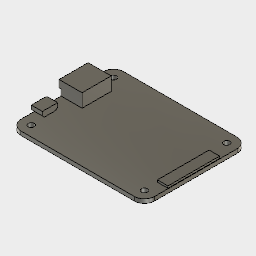
2218 HDMI TPF401 Breakout (Autodesk Fusion 360 design; units mm, degrees)
Autodesk Fusion 360 part; units mm, degrees
sketch "PCB" plane through (0, 0, 0) normal (0, 0, 1) x (1, 0, 0)
  line L0 (0, 0) -> (66.04, 0)
  line L1 (66.04, 0) -> (66.04, 50.8)
  line L2 (66.04, 50.8) -> (0, 50.8)
  line L3 (0, 50.8) -> (0, 0)
  circle A0 centre (5.08, 45.72) radius 1.5
  line L4 (33.02, 50.8) -> (33.02, 0) construction
  line L5 (0, 25.4) -> (66.04, 25.4) construction
  circle A1 centre (60.96, 45.72) radius 1.5
  circle A2 centre (5.08, 5.08) radius 1.5
  circle A3 centre (60.96, 5.08) radius 1.5
  dimension "d1" = 66.04
  dimension "d2" = 50.8
  dimension "d3" = 3
  dimension "d4" = 5.08
  dimension "d5" = 45.72
  measures "d1" distance of L1.end L2.end
  measures "d2" distance of L0.end L1.end
  measures "d3" diameter of A0
  measures "d4" distance of L3 A0.centre
  measures "d5" distance of L0 A0.centre
extrude "Extrude1" add sketch "PCB" along normal blind 2 makes body 1
fillet "Fillet1" radius 5.08 4 edges at (66.04, 0, 1) (0, 0, 1) (0, 50.8, 1) (66.04, 50.8, 1) on bodies 1
sketch "hdmi usb" plane through (0, 0, 2) normal (0, 0, 1) x (-1, 0, 0)
  arc A0 (-66.04, -45.72) -> (-60.96, -50.8) centre (-60.96, -45.72) ccw
  line L0 (-60.96, -50.8) -> (-5.08, -50.8)
  arc A1 (-5.08, -50.8) -> (0, -45.72) centre (-5.08, -45.72) ccw
  line L1 (0, -45.72) -> (0, -5.08)
  arc A2 (0, -5.08) -> (-5.08, 0) centre (-5.08, -5.08) ccw
  line L2 (-5.08, 0) -> (-60.96, 0)
  arc A3 (-60.96, 0) -> (-66.04, -5.08) centre (-60.96, -5.08) ccw
  line L3 (-66.04, -5.08) -> (-66.04, -45.72)
  circle A4 centre (-60.96, -5.08) radius 1.5
  circle A5 centre (-60.96, -45.72) radius 1.5
  circle A6 centre (-5.08, -45.72) radius 1.5
  circle A7 centre (-5.08, -5.08) radius 1.5
  line L4 (1, -39.24) -> (-10.4, -39.24)
  line L5 (-10.4, -39.24) -> (-10.4, -24.84)
  line L6 (-10.4, -24.84) -> (1, -24.84)
  line L7 (1, -24.84) -> (1, -39.24)
  line L8 (0.6, -18.34) -> (-4.9, -18.34)
  line L9 (-4.9, -18.34) -> (-4.9, -10.74)
  line L10 (-4.9, -10.74) -> (0.6, -10.74)
  line L11 (0.6, -10.74) -> (0.6, -18.34)
  dimension "d9" = 11.4
  dimension "d10" = 14.4
  dimension "d11" = 1
  dimension "d12" = 11.56
  dimension "d13" = 5.5
  dimension "d14" = 7.6
  dimension "d15" = 0.6
  dimension "d16" = 6.5
  measures "d9" distance of L4.start L4.end
  measures "d10" distance of L4.start L6.end
  measures "d11" distance of L1 L7
  measures "d12" distance of L0 L4
  measures "d13" distance of L8.start L8.end
  measures "d14" distance of L8.start L10.end
  measures "d15" distance of L1 L11
  measures "d16" distance of L6 L8
extrude "Extrude2" add sketch "hdmi usb" along normal blind 5.6 from surface at 1 separate body contours L1 L4 L5 L6 | L1 L4 L6 L7 makes body 2
chamfer "Chamfer1" distance 2 angle 45 2 edges at (4.7, 24.84, 3) (4.7, 39.24, 3) on bodies 2
extrude "Extrude3" add sketch "hdmi usb" along normal blind 2.9 separate body contours L1 L8 L10 L11 | L1 L8 L9 L10 makes body 3
chamfer "Chamfer2" distance 1 angle 45 2 edges at (2.15, 18.34, 2) (2.15, 10.74, 2) on bodies 3
sketch "hdmi 2" plane through (0, 0, 3) normal (0, 0, -1) x (1, 0, 0)
  line L0 (-1, -37.24) -> (10.4, -37.24)
  line L1 (10.4, -37.24) -> (10.4, -26.84)
  line L2 (10.4, -26.84) -> (-1, -26.84)
  line L3 (-1, -26.84) -> (-1, -37.24)
  line L4 (0, -45.72) -> (0, -5.08)
  line L5 (-1, -24.84) -> (10.4, -24.84)
  line L6 (10.4, -24.84) -> (10.4, -39.24)
  line L7 (10.4, -39.24) -> (-1, -39.24)
  line L8 (-1, -39.24) -> (-1, -24.84)
extrude "Extrude4" add sketch "hdmi 2" along normal blind 1 contours L0 L1 L2 L4 L6 bodies 2
extrude "Extrude5" add sketch "hdmi 2" along normal blind -2.5 and the other way blind -1 contours L0 L4 L6 L7 | L2 L4 L5 L6 bodies 2
sketch "Sketch4" plane through (0, 0, 2) normal (0, 0, 1) x (-1, 0, 0)
  arc A0 (-66.04, -45.72) -> (-60.96, -50.8) centre (-60.96, -45.72) ccw
  line L0 (-60.96, -50.8) -> (-5.08, -50.8)
  arc A1 (-5.08, -50.8) -> (0, -45.72) centre (-5.08, -45.72) ccw
  line L1 (0, -45.72) -> (0, -5.08)
  arc A2 (0, -5.08) -> (-5.08, 0) centre (-5.08, -5.08) ccw
  line L2 (-5.08, 0) -> (-60.96, 0)
  arc A3 (-60.96, 0) -> (-66.04, -5.08) centre (-60.96, -5.08) ccw
  line L3 (-66.04, -5.08) -> (-66.04, -45.72)
  circle A4 centre (-60.96, -5.08) radius 1.5
  circle A5 centre (-60.96, -45.72) radius 1.5
  circle A6 centre (-5.08, -45.72) radius 1.5
  circle A7 centre (-5.08, -5.08) radius 1.5
  line L4 (-60.64, -37.3) -> (-65.84, -37.3)
  line L5 (-65.84, -37.3) -> (-65.84, -11.8)
  line L6 (-65.84, -11.8) -> (-60.64, -11.8)
  line L7 (-60.64, -11.8) -> (-60.64, -37.3)
  line L8 (-60.64, -24.55) -> (-65.84, -24.55) construction
  dimension "d30" = 25.5
  dimension "d31" = 24.55
  dimension "d32" = 0.2
  dimension "d33" = 5.2
  measures "d30" distance of L4.end L5.end
  measures "d31" distance of L2 L8
  measures "d32" distance of L3 L5
  measures "d33" distance of L4.start L4.end
extrude "Extrude6" add sketch "Sketch4" along normal blind 1 separate body contours L4 L5 L6 L7 makes body 4
